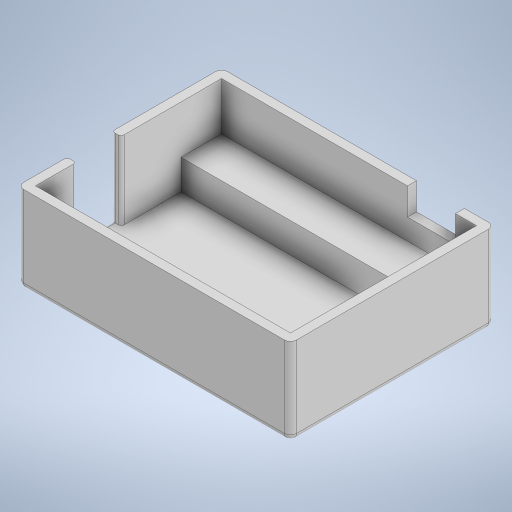
# Autodesk Inventor part: Glove Case
Saved by Autodesk Inventor 2023 (Build 270158000, 158)
## iProperties
Created: 2023-08-02
Part Number: Glove Case
Material: Generic
Document SubType Name: Modeling
Designer: campstudent
Density: 1 g/cm^3
Appearance: Default
Author: campstudent
Autodesk Inventor part; units mm, degrees
ref_plane "YZ Plane" through (0, 0, 0) normal (1, 0, 0) x (0, 1, 0)
ref_plane "XZ Plane" through (0, 0, 0) normal (0, 1, 0) x (-1, 0, 0)
ref_plane "XY Plane" through (0, 0, 0) normal (0, 0, 1) x (1, 0, 0)
sketch "Sketch1" plane through (0, 0, 0) normal (0, 1, 0) x (-1, 0, 0)
  line L0 (0, 0) -> (91, 0)
  line L1 (91, 0) -> (91, -68)
  line L2 (91, -68) -> (0, -68)
  line L3 (0, -68) -> (0, 0)
  line L4 (88, -3) -> (3, -3)
  line L5 (3, -3) -> (3, -65)
  line L6 (3, -65) -> (88, -65)
  line L7 (88, -65) -> (88, -3)
  dimension "d0" = 91
  dimension "d1" = 68
  dimension "d2" = 62
  dimension "d3" = 85
  dimension "d4" = 3
  dimension "d5" = 3
  constraints: 16 end point, 4 parallel, 2 horizontal, 2 perpendicular
  measures "d0" distance of L1.end L2.end
  measures "d1" distance of L0.end L1.end
  measures "d2" distance of L6.end L4.start
  measures "d3" distance of L5.end L6.end
  measures "d4" distance between parallel lines of L1 L7
  measures "d5" distance between parallel lines of L2 L6
extrude "Extrusion1" add sketch "Sketch1" along normal blind 29 contours L0 L1 L2 L3 | L7 L6 L5 L4
sketch "Sketch2" plane through (0, 29, 0) normal (0, 1, 0) x (1, 0, 0)
  line L0 (-88, 16.5) -> (-3, 16.5)
  line L1 (-3, 16.5) -> (-3, 51.5)
  line L2 (-3, 51.5) -> (-88, 51.5)
  line L3 (-88, 51.5) -> (-88, 16.5)
  line L4 (-91, 68) -> (-91, 0) projected
  line L5 (0, 68) -> (-91, 68) projected
  point P0 (0, 0)
  dimension "d8" = 85
  dimension "d9" = 35
  dimension "d10" = 3
  dimension "d11" = 16.5
  constraints: 8 end point, 2 parallel, 1 horizontal, 1 perpendicular
  measures "d8" distance of L2.end L1.end
  measures "d9" distance of L1.end L0.end
  measures "d10" distance between parallel lines of L4 L3
  measures "d11" distance between parallel lines of L5 L2
extrude "Extrusion2" cut sketch "Sketch2" against normal blind 26
sketch "Sketch3" plane through (0, 29, 0) normal (0, 1, 0) x (1, 0, 0)
  line L0 (-88, 3) -> (-3, 3)
  line L1 (-3, 3) -> (-3, 65)
  line L2 (-3, 65) -> (-88, 65)
  line L3 (-88, 65) -> (-88, 3)
  line L4 (-91, 68) -> (-91, 0) projected
  line L5 (0, 68) -> (-91, 68) projected
  point P0 (0, 0)
  point P1 (-45.5, 68)
  dimension "d14" = 62
  dimension "d15" = 85
  dimension "d16" = 3
  dimension "d17" = 3
  constraints: 8 end point, 2 parallel, 1 horizontal, 1 midpoint, 1 perpendicular
  measures "d14" distance of L2.end L0.start
  measures "d15" distance of L1.end L2.end
  measures "d16" distance between parallel lines of L4 L3
  measures "d17" distance from line of point (-45.5, 68) L2
extrude "Extrusion3" cut sketch "Sketch3" against normal blind 16
sketch "Sketch4" plane through (0, 0, -68) normal (0, 0, -1) x (-1, 0, 0)
  line L0 (88, 29) -> (3, 29) projected
  line L1 (10, 29) -> (26, 29)
  line L2 (26, 29) -> (26, 20)
  line L3 (26, 20) -> (10, 20)
  line L4 (10, 20) -> (10, 29)
  line L5 (0, 0) -> (0, 29) projected
  point P0 (26, 29)
  dimension "d20" = 16
  dimension "d21" = 9
  dimension "d22" = 10
  constraints: 8 end point, 2 parallel, 1 horizontal, 1 perpendicular, 1 point on line
  measures "d20" distance of L2.end L3.end
  measures "d21" distance of L1.end L2.end
  measures "d22" distance between parallel lines of L5 L4
extrude "Extrusion4" cut sketch "Sketch4" against normal blind 4
sketch "Sketch5" plane through (0, 13, 0) normal (0, 1, 0) x (1, 0, 0)
  circle A0 centre (-75, 7.5) radius 0.95
  line L0 (-88, 3) -> (-88, 65) projected
  line L1 (-3, 3) -> (-88, 3) projected
  circle A1 centre (-10.5, 61.5) radius 0.95
  line L2 (-88, 65) -> (-26, 65) projected
  line L3 (-3, 65) -> (-3, 3) projected
  point P0 (0, 0)
  dimension "d25" = 1.9
  dimension "d26" = 13
  dimension "d27" = 4.5
  dimension "d28" = 1.9
  dimension "d29" = 3.5
  dimension "d30" = 7.5
  constraints: 2 centre point
  measures "d25" diameter of A0
  measures "d26" distance from line of L0 A0.centre
  measures "d27" distance from line of L1 A0.centre
  measures "d28" diameter of A1
  measures "d29" distance from line of A1.centre L2
  measures "d30" distance from line of L3 A1.centre
extrude "Extrusion5" cut sketch "Sketch5" against normal blind 10
fillet "Fillet1" radius 2 8 edges at (0, 14.5, -68) (0, 14.5, 0) (0, 0, -34) (-45.5, 0, -68) (-91, 14.5, -68) (-91, 14.5, 0) (-91, 0, -34) (-45.5, 0, 0)
sketch "Sketch6" plane through (-88, 3, -16.5) normal (1, 0, 0) x (0, 0, -1)
  line L0 (0, 0) -> (15, 0)
  line L1 (15, 0) -> (15, 27)
  line L2 (15, 27) -> (0, 27)
  line L3 (0, 27) -> (0, 0)
  point P0 (-16.5, -3)
  dimension "d34" = 15
  dimension "d35" = 27
  constraints: 8 end point, 2 parallel, 1 horizontal, 1 perpendicular
  measures "d34" distance of L2.end L1.end
  measures "d35" distance of L0.end L1.end
extrude "Extrusion6" cut sketch "Sketch6" against normal blind 10
fillet "Fillet2" radius 1 5 edges at (-88, 16, -31.5) (-91, 16, -31.5) (-91, 16, -16.5) (-88, 21, -16.5) (-91, 3, -24)
body "Solid1"
